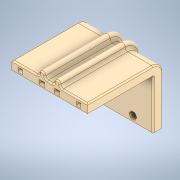
# Autodesk Inventor part: battery mount bracket
Saved by Autodesk Inventor 2022.2 (Build 262287000, 287)
## iProperties
Created: 2022-04-23
Part Number: battery mount bracket
Material: Polyethylene, High Density
Document SubType Name: Modeling
Designer: foriw
Density: 0.952 g/cm^3
Appearance: Smooth - Off-White
Mass: 305.141 g
Surface Area: 723.994 cm^2
Volume: 320.526 cm^3
Author: foriw
Autodesk Inventor part; units mm, degrees
ref_plane "YZ Plane" through (0, 0, 0) normal (1, 0, 0) x (0, 1, 0)
ref_plane "XZ Plane" through (0, 0, 0) normal (0, 1, 0) x (-1, 0, 0)
ref_plane "XY Plane" through (0, 0, 0) normal (0, 0, 1) x (1, 0, 0)
sketch "Sketch1" plane through (0, 0, 0) normal (0, 0, 1) x (1, 0, 0)
  line L0 (27, 27.5) -> (-27, 27.5)
  line L1 (-27, 27.5) -> (-27, -27.5)
  line L2 (-27, -27.5) -> (27, -27.5)
  line L3 (27, -27.5) -> (27, 27.5)
  line L4 (27, 27.5) -> (-27, -27.5) construction
  line L5 (-27, 27.5) -> (27, -27.5) construction
  line L6 (37, -37.5) -> (-37, -37.5)
  line L7 (-37, -37.5) -> (-37, 37.5)
  line L8 (-37, 37.5) -> (37, 37.5)
  line L9 (37, 37.5) -> (37, -37.5)
  line L10 (24.1132, -32.5) -> (21.2265, -27.5)
  line L11 (21.2265, -27.5) -> (24.1132, -22.5)
  line L12 (24.1132, -22.5) -> (29.8868, -22.5)
  line L13 (29.8868, -22.5) -> (32.7735, -27.5)
  line L14 (32.7735, -27.5) -> (29.8868, -32.5)
  line L15 (29.8868, -32.5) -> (24.1132, -32.5)
  line L16 (-29.8868, -32.5) -> (-32.7735, -27.5)
  line L17 (-32.7735, -27.5) -> (-29.8868, -22.5)
  line L18 (-29.8868, -22.5) -> (-24.1132, -22.5)
  line L19 (-24.1132, -22.5) -> (-21.2265, -27.5)
  line L20 (-21.2265, -27.5) -> (-24.1132, -32.5)
  line L21 (-24.1132, -32.5) -> (-29.8868, -32.5)
  line L22 (-24.1132, 32.5) -> (-21.2265, 27.5)
  line L23 (-21.2265, 27.5) -> (-24.1132, 22.5)
  line L24 (-24.1132, 22.5) -> (-29.8868, 22.5)
  line L25 (-29.8868, 22.5) -> (-32.7735, 27.5)
  line L26 (-32.7735, 27.5) -> (-29.8868, 32.5)
  line L27 (-29.8868, 32.5) -> (-24.1132, 32.5)
  line L28 (29.8868, 32.5) -> (32.7735, 27.5)
  line L29 (32.7735, 27.5) -> (29.8868, 22.5)
  line L30 (29.8868, 22.5) -> (24.1132, 22.5)
  line L31 (24.1132, 22.5) -> (21.2265, 27.5)
  line L32 (21.2265, 27.5) -> (24.1132, 32.5)
  line L33 (24.1132, 32.5) -> (29.8868, 32.5)
  line L34 (57.5, -37.5) -> (57.5, 37.5)
  line L35 (57.5, 37.5) -> (37, 37.5)
  line L36 (57.5, -37.5) -> (37, -37.5)
  line L37 (0, -37.5) -> (0, 0) construction
  line L38 (-57.5, -37.5) -> (-57.5, 37.5)
  line L39 (-57.5, 37.5) -> (-37, 37.5)
  line L40 (-57.5, -37.5) -> (-37, -37.5)
  line L41 (57.5, 37.5) -> (57.5, 137.5)
  line L42 (57.5, 137.5) -> (-57.5, 137.5)
  line L43 (-57.5, 137.5) -> (-57.5, 37.5)
  point P0 (27, -32.5)
  point P1 (-27, -32.5)
  point P2 (-27, 32.5)
  dimension "d0" = 54
  dimension "d1" = 55
  dimension "d2" = 10
  dimension "d12" = 10
  dimension "d13" = 10
  dimension "d14" = 10
  dimension "d15" = 10
  dimension "d21" = 115
  dimension "d33" = 100
  constraints: 88 end point, 8 coincident, 6 midpoint, 6 perpendicular, 4 parallel, 3 symmetric about line, 2 horizontal, 2 point on line, 2 vertical, 55 other
  measures "d0" distance of L1.end L2.end
  measures "d1" distance of L0.end L1.end
  measures "d2" distance between parallel lines of L2 L6
  measures "d12" distance between parallel lines of L15 L12
  measures "d13" distance between parallel lines of L19 L16
  measures "d14" distance between parallel lines of L33 L30
  measures "d15" distance from line of point (-27, 32.5) L24
  measures "d21" distance of L38.start L34.start
  measures "d33" distance of L34.end L41.end
extrude "Extrusion1" add sketch "Sketch1" against normal blind 15 contours L3 L30 L31 L0 | L0 L32 L33 L28 L29 L30 L3 | L31 L30 L3 L12 L11 L2 L19 L18 L1 L24 L23 L0 | L23 L24 L1 L0 | L0 L1 L24 L25 L26 L27 L22 | L12 L13 L14 L15 L10 L2 L3 | L3 L2 L11 L12 | L18 L19 L2 L1 | L1 L2 L20 L21 L16 L17 L18 | L6 L7 L8 L9 | L8 L39 L43 L42 L41 L35
hole "Hole1" at (27, 27.5, 0) at (-27, 27.5, 0) at (-27, -27.5, 0) at (27, -27.5, 0) direction (0, 0, -1) diameter 7 end through all
extrude "Extrusion2" cut sketch "Sketch1" against normal blind 8 contours L3 L30 L31 L0 | L0 L32 L33 L28 L29 L30 L3 | L23 L24 L1 L0 | L0 L1 L24 L25 L26 L27 L22 | L12 L13 L14 L15 L10 L2 L3 | L3 L2 L11 L12 | L18 L19 L2 L1 | L1 L2 L20 L21 L16 L17 L18
extrude "Extrusion3" add sketch "Sketch1" against normal blind 15 contours L9 L35 L34 L36 | L40 L38 L39 L7
sketch "Sketch2" plane through (-37, -37.5, 0) normal (0, -1, 0) x (1, 0, 0)
  line L0 (94.5, 0) -> (94.5, -15)
  line L1 (94.5, -10.6722) -> (-20.5, -10.6722)
  line L2 (-20.5, 0) -> (-20.5, -15)
  line L3 (-20.5, -6.6722) -> (94.5, -6.6722)
  line L4 (84.5, -15) -> (84.5, 0)
  line L5 (78.5, 0) -> (78.5, -15)
  line L6 (-20.5, -15) -> (94.5, -15)
  line L7 (37, -15) -> (37, 0) construction
  line L8 (-10.5, -15) -> (-10.5, 0)
  line L9 (-4.5, 0) -> (-4.5, -15)
  line L10 (-20.5, 0) -> (94.5, 0)
  line L11 (0, -15) -> (74, -15)
  line L12 (52.5, -15) -> (52.5, 0)
  line L13 (44.5, -15) -> (44.5, 0)
  line L14 (94.5, 0) -> (-20.5, 0)
  line L15 (21.5, -15) -> (21.5, 0)
  line L16 (29.5, -15) -> (29.5, 0)
  line L17 (52.5, -15) -> (44.5, -15)
  line L18 (44.5, -15) -> (44.5, -23)
  line L19 (44.5, -23) -> (52.5, -23)
  line L20 (52.5, -23) -> (52.5, -15)
  line L21 (29.5, -15) -> (21.5, -15)
  line L22 (21.5, -15) -> (21.5, -23)
  line L23 (21.5, -23) -> (29.5, -23)
  line L24 (29.5, -23) -> (29.5, -15)
  point P0 (-4.5, -10.6722)
  point P1 (-4.5, -6.6722)
  point P2 (-10.5, -6.6722)
  point P3 (-10.5, -10.6722)
  point P4 (78.5, -6.6722)
  point P5 (78.5, -10.6722)
  point P6 (84.5, -10.6722)
  point P7 (84.5, -6.6722)
  point P8 (-20.5, 0)
  point P9 (94.5, 0)
  point P10 (74, 0)
  point P11 (0, 0)
  point P12 (52.5, -7.5)
  point P13 (29.5, -10.6722)
  point P14 (29.5, -6.6722)
  point P15 (21.5, -6.6722)
  point P16 (21.5, -10.6722)
  point P17 (44.5, -6.6722)
  point P18 (44.5, -10.6722)
  point P19 (52.5, -10.6722)
  point P20 (52.5, -6.6722)
  dimension "d18" = 4
  dimension "d19" = 6
  dimension "d20" = 10
  dimension "d26" = 8
  dimension "d27" = 42
  dimension "d36" = 8
  dimension "d37" = 8
  constraints: 48 end point, 8 symmetric about line, 7 point on line, 5 vertical, 4 horizontal, 4 parallel, 3 coincident, 2 midpoint, 2 perpendicular, 4 other
  measures "d18" distance between parallel lines of L1 L3
  measures "d19" distance between parallel lines of L5 L4
  measures "d20" distance between parallel lines of L0 L4
  measures "d26" distance from line of point (52.5, -7.5) L13
  measures "d27" distance between parallel lines of L12 L0
  measures "d36" distance of L13.start L18.end
  measures "d37" distance of L15.start L22.end
extrude "Extrusion6" add sketch "Sketch2" against normal up to surface (175 mm away) contours L20 L19 L18 L6 | L24 L23 L22 L6
extrude "Extrusion4" cut sketch "Sketch2" against normal through all contours L4 L1 L5 L3 | L12 L1 L13 L3 | L16 L1 L15 L3 | L9 L1 L8 L3
ref_plane "Work Plane1" through (0, 0, -38.25) normal (0, 0, -1) x (-1, 0, 0)
bend part "Bend Part1" radius 0.5 angle 90 line through (-37, 37.5, 0) along (1, 0, 0) centre toward (0, 0, 1) moving side (0, 1, 0) both sides no
fillet "Fillet2" radius 4 12 edges at (7.5, 0, -15) (7.5, 53, 50.1073) (7.5, 48.4602, -10.4602) (7.5, 61, 50.1073) (7.5, 0, -23) (7.5, 54.117, -16.117) (15.5, 61, 50.1073) (15.5, 0, -23) (15.5, 54.117, -16.117) (15.5, 53, 50.1073) (15.5, 0, -15) (15.5, 48.4602, -10.4602)
fillet "Fillet3" radius 4 12 edges at (-15.5, 54.117, -16.117) (-15.5, 61, 50.1073) (-15.5, 0, -23) (-7.5, 54.117, -16.117) (-7.5, 61, 50.1073) (-7.5, 0, -23) (-15.5, 48.4602, -10.4602) (-15.5, 53, 50.1073) (-15.5, 0, -15) (-7.5, 48.4602, -10.4602) (-7.5, 53, 50.1073) (-7.5, 0, -15)
chamfer "Chamfer1" distance 2 angle 45 30 edges at (-57.5, 38, 50.1073) (-57.5, 37.8536, 0.1464) (-57.5, 0, 0) (-57.5, 48.4602, -10.4602) (-57.5, 53, 50.1073) (-57.5, 0, -15) (57.5, 38, 50.1073) (57.5, 37.8536, 0.1464) (57.5, 0, 0) (57.5, 53, 50.1073) (57.5, 48.4602, -10.4602) (57.5, 0, -15) (0, 38, 99.7146) (38.4999, 53, 99.7146) (15.5, 57, 99.7146) (16.6715, 54.1715, 99.7146) (7.5, 57, 99.7146) (14.3285, 59.8285, 99.7146) (11.5, 61, 99.7146) (8.6715, 59.8285, 99.7146) (6.3285, 54.1715, 99.7146) (0, 53, 99.7146) (-7.5, 57, 99.7146) (-6.3285, 54.1715, 99.7146) (-15.5, 57, 99.7146) (-14.3285, 59.8285, 99.7146) (-11.5, 61, 99.7146) (-8.6715, 59.8285, 99.7146) (-16.6715, 54.1715, 99.7146) (-38.5, 53, 99.7146)
fillet "Fillet4" radius 3 8 edges at (11.5, -37.5, -6.6722) (-11.5, -37.5, -6.6722) (-44.5, -37.5, -6.6722) (44.5, -37.5, -6.6722) (44.5, 44.6722, 99.7146) (11.5, 44.6722, 99.7146) (-11.5, 44.6722, 99.7146) (-44.5, 44.6722, 99.7146)
chamfer "Chamfer2" distance 2 angle 45 40 edges at (57.5, -37.5, -7.5) (37.4999, -37.5, -15) (16.6715, -37.5, -16.1715) (15.5, -37.5, -19) (7.5, -37.5, -19) (14.3285, -37.5, -21.8285) (8.6715, -37.5, -21.8285) (11.5, -37.5, -23) (6.3285, -37.5, -16.1715) (0, -37.5, -15) (-7.5, -37.5, -19) (-6.3285, -37.5, -16.1715) (-15.5, -37.5, -19) (-14.3285, -37.5, -21.8285) (-11.5, -37.5, -23) (-8.6715, -37.5, -21.8285) (-16.6715, -37.5, -16.1715) (-37.4999, -37.5, -15) (0, -37.5, 0) (-57.5, -37.5, -7.5) (-47.5, -37.5, -5.1722) (-47.5, -37.5, -8.6722) (-44.5, -37.5, -10.6722) (-41.5, -37.5, -5.1722) (-41.5, -37.5, -8.6722) (-15.5, -37.5, -5.1722) (-15.5, -37.5, -8.6722) (-11.5, -37.5, -10.6722) (-7.5, -37.5, -5.1722) (-7.5, -37.5, -8.6722) (7.5, -37.5, -5.1722) (7.5, -37.5, -8.6722) (11.5, -37.5, -10.6722) (15.5, -37.5, -5.1722) (15.5, -37.5, -8.6722) (41.5, -37.5, -5.1722) (41.5, -37.5, -8.6722) (44.5, -37.5, -10.6722) (47.5, -37.5, -5.1722) (47.5, -37.5, -8.6722)
equation "\"d13\" = d12"
equation "\"d14\" = d12"
equation "\"d15\" = d12"
body "Solid1"
